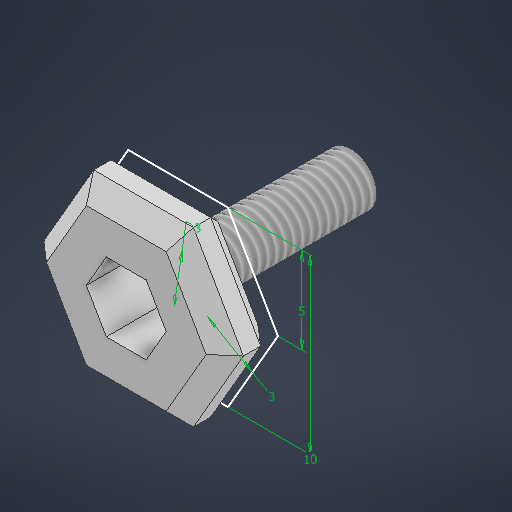
# Autodesk Inventor part: Parafuso
Saved by Autodesk Inventor 2026.2 (Build 302298010, 298A)
## iProperties
Created: 2026-04-17
Part Number: Parafuso
Material: Generic
Document SubType Name: Modeling
Designer: mrcm
Density: 1 g/cm^3
Appearance: Default
Author: mrcm
Autodesk Inventor part; units mm, degrees
ref_plane "YZ Plane" through (0, 0, 0) normal (1, 0, 0) x (0, 1, 0)
ref_plane "XZ Plane" through (0, 0, 0) normal (0, 1, 0) x (-1, 0, 0)
ref_plane "XY Plane" through (0, 0, 0) normal (0, 0, 1) x (1, 0, 0)
sketch "Sketch1" plane through (0, 0, 0) normal (0, 0, 1) x (1, 0, 0)
  line L0 (-2.8868, 5) -> (2.8868, 5)
  line L1 (2.8868, 5) -> (5.7735, 0)
  line L2 (5.7735, 0) -> (2.8868, -5)
  line L3 (2.8868, -5) -> (-2.8868, -5)
  line L4 (-2.8868, -5) -> (-5.7735, 0)
  line L5 (-5.7735, 0) -> (-2.8868, 5)
  circle A0 centre (0, 0) radius 1.5
  line L6 (1.1547, -2) -> (2.3094, 0)
  line L7 (2.3094, 0) -> (1.1547, 2)
  line L8 (1.1547, 2) -> (-1.1547, 2)
  line L9 (-1.1547, 2) -> (-2.3094, 0)
  line L10 (-2.3094, 0) -> (-1.1547, -2)
  line L11 (-1.1547, -2) -> (1.1547, -2)
  dimension "d0" = 3
  dimension "d1" = 10
  dimension "d2" = 5
  dimension "d12" = 3
  constraints: 24 end point, 2 coincident, 1 centre point, 18 other
  measures "d0" diameter of A0
  measures "d1" distance between parallel lines of L3 L0
  measures "d2" vertical distance of L0.end L1.end
  measures "d12" distance between parallel lines of L6 L2
extrude "Extrusion1" add sketch "Sketch1" along normal blind 3 contours L0 L1 L2 L3 L4 L5 | A0 | L11 L10 L9 L8 L7 L6
extrude "Extrusion2" add sketch "Sketch1" against normal blind 10 contours A0
thread "Thread1" size "M3x0.5" class "6g" standard "ANSI Metric M Profile" full length
chamfer "Chamfer1" distance 1 angle 45 12 edges at (4.3301, -2.5, 0) (4.3301, 2.5, 0) (0, -5, 0) (-4.3301, -2.5, 0) (-4.3301, 2.5, 0) (0, 5, 0) (0, 5, 3) (-4.3301, 2.5, 3) (-4.3301, -2.5, 3) (0, -5, 3) (4.3301, -2.5, 3) (4.3301, 2.5, 3)
extrude "Extrusion3" cut sketch "Sketch1" along normal blind 10 contours A0 | L11 L10 L9 L8 L7 L6
body "Solid1"
